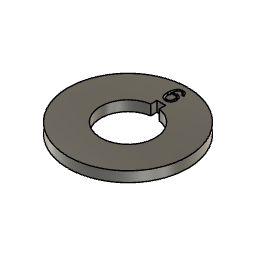
DIN Cover v1.0 (Autodesk Fusion 360 design; units mm, degrees)
Autodesk Fusion 360 part; units mm, degrees
sketch "Sketch1" plane through (0, 0, 0) normal (0, 0, 1) x (1, 0, 0)
  circle A0 centre (0, 0) radius 17.5
  line L0 (0, 0) -> (0, 8) construction
  line L1 (0, 8) -> (0, 9.75) construction
  line L2 (0, 9.75) -> (1.25, 9.75)
  line L3 (0, 9.75) -> (-1.25, 9.75)
  line L4 (-1.25, 9.75) -> (-1.25, 7.9017)
  line L5 (1.25, 9.75) -> (1.25, 7.9017)
  arc A1 (-1.25, 7.9017) -> (1.25, 7.9017) centre (0, 0) ccw
  dimension "d1" = 16
  dimension "d2" = 35
  dimension "d3" = 1.75
  dimension "d4" = 1.25
  dimension "d5" = 1.25
  constraint coincident A0.centre L0.start
  constraint vertical L0
  constraint parallel L0 L1
  constraint perpendicular L1 L2
  constraint perpendicular L1 L3
  constraint perpendicular L3 L4
  constraint perpendicular L2 L5
  measures "d1" diameter of A1
  measures "d2" diameter of A0
  measures "d3" distance of L0.end L1.end
  measures "d4" distance of L1.end L2.end
  measures "d5" distance of L1.end L3.end
extrude "Extrude1" add sketch "Sketch1" along normal blind 3
sketch "Sketch2" plane through (0, 0, 3) normal (0, 0, 1) x (-1, 0, 0)
  line L0 (1.25, -9.75) -> (-1.25, -9.75)
  line L1 (-1.25, -9.75) -> (-1.25, -7.9017)
  arc A0 (1.25, -7.9017) -> (-1.25, -7.9017) centre (0, 0) ccw
  line L2 (1.25, -7.9017) -> (1.25, -9.75)
  circle A1 centre (0, 0) radius 17.5
  line L3 (0, -9.75) -> (0, -17.5) construction
  line L4 (1.9479, -12.3145) -> (-1.0361, -12.3194) construction
  line L5 (-1.0361, -12.3194) -> (-1.0279, -17.3197) construction
  line L6 (-1.0279, -17.3197) -> (1.9561, -17.3148) construction
  line L7 (1.9561, -17.3148) -> (1.9479, -12.3145) construction
  dimension "d8" = 5
  text T0 "6" font "Arial" height 5 align left top in box 2.984 x 5.0004 at (1.9479, -12.3145) x (-0.999999, -0.001643) y (0.001643, -0.999999) spacing 1 kerned
  constraint midpoint L0 L3.start
  constraint coincident A1 L3.end
  constraint perpendicular L0 L3
extrude "Extrude2" cut sketch "Sketch2" against normal blind 1 text T0
